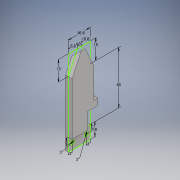
# Autodesk Inventor part: armmodulepart1
Saved by Autodesk Inventor 2018.3 (Build 223284000, 284)
## iProperties
Created: 2019-11-02
Part Number: armmodulepart1
Material: 一般
Document SubType Name: Modeling
Designer: Eiji Nishizawa
Density: 1 g/cm^3
Appearance: 既定
Author: Eiji Nishizawa
Autodesk Inventor part; units mm, degrees
ref_plane "YZ Plane" through (0, 0, 0) normal (1, 0, 0) x (0, 1, 0)
ref_plane "XZ Plane" through (0, 0, 0) normal (0, 1, 0) x (-1, 0, 0)
ref_plane "XY Plane" through (0, 0, 0) normal (0, 0, 1) x (1, 0, 0)
sketch "スケッチ1" plane through (0, 0, 0) normal (1, 0, 0) x (0, 1, 0)
  line L0 (9.2985, 24.3383) -> (-7.3015, 24.3383)
  line L1 (-7.3015, 24.3383) -> (-7.3015, -40.6617)
  line L2 (-7.3015, -40.6617) -> (9.2985, -40.6617)
  line L3 (9.2985, -40.6617) -> (9.2985, 24.3383)
  line L4 (-7.3015, -40.6617) -> (9.2985, -40.6617)
  line L5 (9.2985, -40.6617) -> (9.2985, -30.6617)
  line L6 (9.2985, -30.6617) -> (-7.3015, -30.6617)
  line L7 (-7.3015, -30.6617) -> (-7.3015, -40.6617)
  circle A0 centre (6.2985, -35.6617) radius 1.5
  circle A1 centre (-4.3015, -35.6617) radius 1.5
  line L8 (2.4985, 24.3383) -> (9.2985, 9.3383)
  line L9 (-0.5015, 24.3383) -> (-7.3015, 9.3383)
  point P0 (0, 0)
  dimension "d0" = 16.6
  dimension "d1" = 10
  dimension "d2" = 3
  dimension "d3" = 3
  dimension "d4" = 5
  dimension "d5" = 5
  dimension "d6" = 3
  dimension "d7" = 3
  dimension "d8" = 3
  dimension "d9" = 15
  dimension "d10" = 15
  dimension "d11" = 6.8
  dimension "d12" = 6.8
  dimension "d13" = 40
  constraints: 20 end point, 5 point on line, 4 parallel, 2 centre point, 2 horizontal, 2 perpendicular
  measures "d0" distance of L0.start L0.end
  measures "d1" distance between parallel lines of L2 L6
  measures "d2" distance from line of L3 A0.centre
  measures "d3" distance from line of L1 A1.centre
  measures "d4" distance from line of L6 A1.centre
  measures "d5" distance from line of L6 A0.centre
  measures "d6" diameter of A0
  measures "d7" diameter of A1
  measures "d8" distance of L9.start L8.start
  measures "d9" distance from line of L0 L9.end
  measures "d10" distance from line of L0 L8.end
  measures "d11" distance from line of L1 L9.start
  measures "d12" distance of L0.start L8.start
  measures "d13" distance from line of L6 L8.end
extrude "押し出し1" add sketch "スケッチ1" against normal blind 2 contours L8 L3 L6 L1 L9 L0 | L3 L2 L1 L6
extrude "押し出し2" add sketch "スケッチ1" along normal blind 3 contours L8 L3 L6 L1 L9 L0
sketch "スケッチ2" plane through (-2, 9.2985, -40.6617) normal (0, 1, 0) x (1, 0, 0)
  line L0 (5, -50) -> (5, -10) projected
  line L1 (0, 0) -> (0, -50) projected
  line L2 (5, -10) -> (0, -10)
  line L3 (0, -10) -> (0, -10.7373)
  line L4 (0, -10.7373) -> (5, -10.7373)
  line L5 (5, -10.7373) -> (5, -10)
  line L6 (5, -22.5) -> (0, -22.5)
  line L7 (0, -22.5) -> (0, -27.5)
  line L8 (0, -27.5) -> (5, -27.5)
  line L9 (5, -27.5) -> (5, -22.5)
  point P0 (2, -40.6617)
  dimension "d18" = 12.5
  dimension "d19" = 5
  constraints: 16 end point, 4 parallel, 3 point on line, 2 horizontal, 2 perpendicular
  measures "d18" distance between parallel lines of L2 L6
  measures "d19" distance between parallel lines of L6 L8
extrude "押し出し3" add sketch "スケッチ2" along normal blind 3 contours L8 L1 L6 L0
chamfer "面取り1" distance 5 angle 45 1 edges at (-2, 0.9985, 24.3383)
sketch "スケッチ3" plane through (-2, 9.2985, -40.6617) normal (0, 1, 0) x (1, 0, 0)
  line L0 (5, -50) -> (5, -10) projected
  line L1 (0, -22.5) -> (5, -22.5)
  line L2 (5, -22.5) -> (5, -10)
  line L3 (5, -10) -> (0, -10)
  line L4 (0, -10) -> (0, -22.5)
  point P0 (2, -40.6617)
  constraints: 8 end point, 2 parallel, 1 horizontal, 1 perpendicular
extrude "押し出し4" cut sketch "スケッチ3" against normal blind 5
